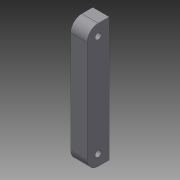
# Autodesk Inventor part: Base
Saved by Autodesk Inventor 2014 SP1 (Build 180222100, 222)
## iProperties
Created: 2014-01-22
Part Number: Base
Material: Generic
Document SubType Name: Modeling
Designer: tom
Density: 1 g/cm^3
Appearance: Default
Author: tom
Autodesk Inventor part; units mm, degrees
ref_plane "YZ Plane" through (0, 0, 0) normal (1, 0, 0) x (0, 1, 0)
ref_plane "XZ Plane" through (0, 0, 0) normal (0, 1, 0) x (-1, 0, 0)
ref_plane "XY Plane" through (0, 0, 0) normal (0, 0, 1) x (1, 0, 0)
sketch "Sketch1" plane through (0, 0, 0) normal (1, 0, 0) x (0, 1, 0)
  circle A0 centre (0, 0) radius 1.778
  circle A1 centre (58.674, 0) radius 1.778
  line L0 (65.024, -6.35) -> (-6.35, -6.35)
  line L1 (-6.35, -6.35) -> (-6.35, 0)
  line L2 (0, 6.35) -> (58.674, 6.35)
  line L3 (65.024, 0) -> (65.024, -6.35)
  arc A2 (0, 6.35) -> (-6.35, 0) centre (0, 0) ccw
  arc A3 (65.024, 0) -> (58.674, 6.35) centre (58.674, 0) ccw
  dimension "d0" = 3.556
  dimension "d1" = 3.556
  dimension "d2" = 58.674
  dimension "d3" = 6.35
  dimension "d4" = 12.7
  dimension "d5" = 6.35
  dimension "d6" = 6.35
  dimension "d8" = 6.35
  constraints: 8 end point, 4 centre point, 4 point on circle, 4 tangent, 2 parallel, 1 coincident, 1 equal radius, 1 horizontal, 1 perpendicular
  measures "d0" diameter of A0
  measures "d1" diameter of A1
  measures "d2" distance of A1.centre A0.centre
  measures "d3" distance from line of L2 point (0, 0)
  measures "d4" distance between parallel lines of L0 L2
  measures "d5" distance from line of L1 point (0, 0)
  measures "d6" distance from line of L3 A1.centre
  measures "d8" radius of A2
extrude "Extrusion1" add sketch "Sketch1" along normal blind 9.525
body "Solid1"
